Autodesk Inventor part; units mm, degrees
(part 2 of 2)
  spline S266 degree 2 poles (0.3678, -0.7093) (0.2402, -0.5675) (0.1065, -0.294) (0.1065, -0.14) knots 0 0 0 1 2 2 2
  spline S267 degree 2 poles (0.1065, -0.14) (0.1065, 0.1355) (0.4712, 0.4475) (0.8176, 0.4475) knots 0 0 0 1 2 2 2
  line L239 (0.8176, 0.4475) -> (2.0352, 0.4475)
  line L240 (2.831, -11.0699) -> (2.831, -12.2328)
  line L241 (2.831, -12.2328) -> (3.536, -12.2328)
  line L242 (3.536, -12.2328) -> (3.536, -11.1185)
  line L243 (3.536, -11.1185) -> (3.8318, -11.1185)
  line L244 (3.8318, -11.1185) -> (3.8318, -12.2328)
  line L245 (3.8318, -12.2328) -> (5.0352, -12.2328)
  line L246 (5.0352, -12.2328) -> (5.0352, -12.565)
  line L247 (5.0352, -12.565) -> (2.5352, -12.565)
  line L248 (2.5352, -12.565) -> (2.5352, -11.0699)
  line L249 (2.5352, -11.0699) -> (2.831, -11.0699)
  line L250 (5.0352, -10.4743) -> (5.0352, -10.7903)
  line L251 (5.0352, -10.7903) -> (3.1592, -10.7903)
  line L252 (3.1592, -10.7903) -> (3.1592, -10.4743)
  line L253 (3.1592, -10.4743) -> (5.0352, -10.4743)
  line L254 (2.8472, -10.452) -> (2.8472, -10.8106)
  line L255 (2.8472, -10.8106) -> (2.519, -10.8106)
  line L256 (2.519, -10.8106) -> (2.519, -10.452)
  line L257 (2.519, -10.452) -> (2.8472, -10.452)
  line L258 (5.0352, -9.6882) -> (5.0352, -10.0043)
  line L259 (5.0352, -10.0043) -> (2.4238, -10.0043)
  line L260 (2.4238, -10.0043) -> (2.4238, -9.6882)
  line L261 (2.4238, -9.6882) -> (5.0352, -9.6882)
  line L262 (5.0352, -8.9022) -> (5.0352, -9.2182)
  line L263 (5.0352, -9.2182) -> (3.1592, -9.2182)
  line L264 (3.1592, -9.2182) -> (3.1592, -8.9022)
  line L265 (3.1592, -8.9022) -> (5.0352, -8.9022)
  line L266 (2.8472, -8.8799) -> (2.8472, -9.2385)
  line L267 (2.8472, -9.2385) -> (2.519, -9.2385)
  line L268 (2.519, -9.2385) -> (2.519, -8.8799)
  line L269 (2.519, -8.8799) -> (2.8472, -8.8799)
  spline S268 degree 2 poles (4.0465, -6.8661) (4.5165, -6.8661) (5.0716, -7.3138) (5.0716, -7.6562) knots 0 0 0 1 2 2 2
  spline S269 degree 2 poles (5.0716, -7.6562) (5.0716, -7.796) (5.0068, -8.0108) (4.94, -8.1222) knots 0 0 0 1 2 2 2
  line L270 (4.94, -8.1222) -> (5.726, -8.1222)
  line L271 (5.726, -8.1222) -> (5.726, -8.4382)
  line L272 (5.726, -8.4382) -> (3.1592, -8.4382)
  line L273 (3.1592, -8.4382) -> (3.1592, -8.1222)
  line L274 (3.1592, -8.1222) -> (3.3557, -8.1222)
  spline S270 degree 2 poles (3.3557, -8.1222) (3.2483, -8.0047) (3.1065, -7.717) (3.1065, -7.5488) knots 0 0 0 1 2 2 2
  spline S271 degree 2 poles (3.1065, -7.5488) (3.1065, -7.2267) (3.617, -6.8661) (4.0465, -6.8661) knots 0 0 0 1 2 2 2
  spline S272 degree 2 poles (4.083, -7.1923) (3.7609, -7.1923) (3.4063, -7.3969) (3.4063, -7.6258) knots 0 0 0 1 2 2 2
  spline S273 degree 2 poles (3.4063, -7.6258) (3.4063, -7.7595) (3.5259, -8.0108) (3.6191, -8.1222) knots 0 0 0 1 2 2 2
  line L275 (3.6191, -8.1222) -> (4.6847, -8.1222)
  spline S274 degree 2 poles (4.6847, -8.1222) (4.7434, -7.9986) (4.788, -7.8223) (4.788, -7.7089) knots 0 0 0 1 2 2 2
  spline S275 degree 2 poles (4.788, -7.7089) (4.788, -7.4638) (4.4274, -7.1923) (4.083, -7.1923) knots 0 0 0 1 2 2 2
  line L276 (5.0352, -4.984) -> (5.0352, -5.3993)
  line L277 (5.0352, -5.3993) -> (4.1296, -6.0962)
  line L278 (4.1296, -6.0962) -> (4.2511, -6.2219)
  line L279 (4.2511, -6.2219) -> (5.0352, -6.2219)
  line L280 (5.0352, -6.2219) -> (5.0352, -6.5379)
  line L281 (5.0352, -6.5379) -> (2.4238, -6.5379)
  line L282 (2.4238, -6.5379) -> (2.4238, -6.2219)
  line L283 (2.4238, -6.2219) -> (3.9513, -6.2219)
  line L284 (3.9513, -6.2219) -> (3.1592, -5.4804)
  line L285 (3.1592, -5.4804) -> (3.1592, -5.0873)
  line L286 (3.1592, -5.0873) -> (3.9432, -5.8572)
  line L287 (3.9432, -5.8572) -> (5.0352, -4.984)
  spline S276 degree 2 poles (4.0972, -3.2843) (4.5712, -3.2843) (5.0879, -3.7401) (5.0879, -4.121) knots 0 0 0 1 2 2 2
  spline S277 degree 2 poles (5.0879, -4.121) (5.0879, -4.512) (4.555, -4.9597) (4.0972, -4.9597) knots 0 0 0 1 2 2 2
  spline S278 degree 2 poles (4.0972, -4.9597) (3.6272, -4.9597) (3.1065, -4.4978) (3.1065, -4.121) knots 0 0 0 1 2 2 2
  spline S279 degree 2 poles (3.1065, -4.121) (3.1065, -3.7401) (3.6251, -3.2843) (4.0972, -3.2843) knots 0 0 0 1 2 2 2
  spline S280 degree 2 poles (4.0972, -3.6104) (3.7325, -3.6104) (3.378, -3.8758) (3.378, -4.121) knots 0 0 0 1 2 2 2
  spline S281 degree 2 poles (3.378, -4.121) (3.378, -4.3661) (3.7325, -4.6335) (4.0972, -4.6335) knots 0 0 0 1 2 2 2
  spline S282 degree 2 poles (4.0972, -4.6335) (4.4517, -4.6335) (4.8164, -4.3661) (4.8164, -4.121) knots 0 0 0 1 2 2 2
  spline S283 degree 2 poles (4.8164, -4.121) (4.8164, -3.8779) (4.4578, -3.6104) (4.0972, -3.6104) knots 0 0 0 1 2 2 2
  line L288 (3.1592, -0.687) -> (5.0352, -1.1631)
  line L289 (5.0352, -1.1631) -> (5.0352, -1.4548)
  line L290 (5.0352, -1.4548) -> (3.5887, -1.9127)
  line L291 (3.5887, -1.9127) -> (5.0352, -2.3685)
  line L292 (5.0352, -2.3685) -> (5.0352, -2.6582)
  line L293 (5.0352, -2.6582) -> (3.1592, -3.1384)
  line L294 (3.1592, -3.1384) -> (3.1592, -2.8102)
  line L295 (3.1592, -2.8102) -> (4.6118, -2.4779)
  line L296 (4.6118, -2.4779) -> (3.1592, -2.0343)
  line L297 (3.1592, -2.0343) -> (3.1592, -1.7729)
  line L298 (3.1592, -1.7729) -> (4.6118, -1.3171)
  line L299 (4.6118, -1.3171) -> (3.1592, -1.0051)
  line L300 (3.1592, -1.0051) -> (3.1592, -0.687)
  spline S284 degree 2 poles (5.0797, 0.097) (5.0797, -0.0914) (4.9785, -0.4176) (4.9217, -0.5249) knots 0 0 0 1 2 2 2
  line L301 (4.9217, -0.5249) -> (4.5672, -0.5249)
  line L302 (4.5672, -0.5249) -> (4.5672, -0.5087)
  spline S285 degree 2 poles (4.5672, -0.5087) (4.5996, -0.4682) (4.6766, -0.3588) (4.7191, -0.2676) knots 0 0 0 1 2 2 2
  spline S286 degree 2 poles (4.7191, -0.2676) (4.7576, -0.1886) (4.8144, 0.0059) (4.8144, 0.1092) knots 0 0 0 1 2 2 2
  spline S287 degree 2 poles (4.8144, 0.1092) (4.8144, 0.1841) (4.7799, 0.3563) (4.7515, 0.3969) knots 0 0 0 1 2 2 2
  spline S288 degree 2 poles (4.7515, 0.3969) (4.7131, 0.4556) (4.6259, 0.5083) (4.5368, 0.5083) knots 0 0 0 1 2 2 2
  spline S289 degree 2 poles (4.5368, 0.5083) (4.4254, 0.5083) (4.3099, 0.3867) (4.2714, 0.2307) knots 0 0 0 1 2 2 2
  spline S290 degree 2 poles (4.2714, 0.2307) (4.2572, 0.17) (4.2167, -0.0245) (4.1944, -0.1076) knots 0 0 0 1 2 2 2
  spline S291 degree 2 poles (4.1944, -0.1076) (4.1316, -0.3223) (3.8723, -0.5168) (3.6879, -0.5168) knots 0 0 0 1 2 2 2
  spline S292 degree 2 poles (3.6879, -0.5168) (3.4327, -0.5168) (3.1146, -0.1339) (3.1146, 0.1821) knots 0 0 0 1 2 2 2
  spline S293 degree 2 poles (3.1146, 0.1821) (3.1146, 0.3381) (3.1916, 0.6542) (3.2503, 0.7615) knots 0 0 0 1 2 2 2
  line L303 (3.2503, 0.7615) -> (3.5887, 0.7615)
  line L304 (3.5887, 0.7615) -> (3.5887, 0.7453)
  spline S294 degree 2 poles (3.5887, 0.7453) (3.4914, 0.6238) (3.38, 0.328) (3.38, 0.176) knots 0 0 0 1 2 2 2
  spline S295 degree 2 poles (3.38, 0.176) (3.38, 0.02) (3.5117, -0.1947) (3.6434, -0.1947) knots 0 0 0 1 2 2 2
  spline S296 degree 2 poles (3.6434, -0.1947) (3.7629, -0.1947) (3.8784, -0.0671) (3.9148, 0.0747) knots 0 0 0 1 2 2 2
  spline S297 degree 2 poles (3.9148, 0.0747) (3.9331, 0.1436) (3.9695, 0.3179) (3.9918, 0.4131) knots 0 0 0 1 2 2 2
  spline S298 degree 2 poles (3.9918, 0.4131) (4.0445, 0.6197) (4.2856, 0.8304) (4.4943, 0.8304) knots 0 0 0 1 2 2 2
  spline S299 degree 2 poles (4.4943, 0.8304) (4.6158, 0.8304) (4.8306, 0.7352) (4.9096, 0.642) knots 0 0 0 1 2 2 2
  spline S300 degree 2 poles (4.9096, 0.642) (4.9926, 0.5427) (5.0797, 0.2895) (5.0797, 0.097) knots 0 0 0 1 2 2 2
  line L305 (5.0352, 2.6781) -> (5.0352, 2.2627)
  line L306 (5.0352, 2.2627) -> (4.1296, 1.5658)
  line L307 (4.1296, 1.5658) -> (4.2511, 1.4402)
  line L308 (4.2511, 1.4402) -> (5.0352, 1.4402)
  line L309 (5.0352, 1.4402) -> (5.0352, 1.1242)
  line L310 (5.0352, 1.1242) -> (2.4238, 1.1242)
  line L311 (2.4238, 1.1242) -> (2.4238, 1.4402)
  line L312 (2.4238, 1.4402) -> (3.9513, 1.4402)
  line L313 (3.9513, 1.4402) -> (3.1592, 2.1817)
  line L314 (3.1592, 2.1817) -> (3.1592, 2.5747)
  line L315 (3.1592, 2.5747) -> (3.9432, 1.8049)
  line L316 (3.9432, 1.8049) -> (5.0352, 2.6781)
  line L317 (5.0352, 3.1582) -> (5.0352, 2.8422)
  line L318 (5.0352, 2.8422) -> (3.1592, 2.8422)
  line L319 (3.1592, 2.8422) -> (3.1592, 3.1582)
  line L320 (3.1592, 3.1582) -> (5.0352, 3.1582)
  line L321 (2.8472, 3.1805) -> (2.8472, 2.8219)
  line L322 (2.8472, 2.8219) -> (2.519, 2.8219)
  line L323 (2.519, 2.8219) -> (2.519, 3.1805)
  line L324 (2.519, 3.1805) -> (2.8472, 3.1805)
  line L325 (10.2664, -10.4256) -> (10.2664, -10.8571)
  line L326 (10.2664, -10.8571) -> (9.2716, -11.6472)
  line L327 (9.2716, -11.6472) -> (9.2716, -12.0281)
  line L328 (9.2716, -12.0281) -> (10.2664, -12.0281)
  line L329 (10.2664, -12.0281) -> (10.2664, -12.3604)
  line L330 (10.2664, -12.3604) -> (7.7664, -12.3604)
  line L331 (7.7664, -12.3604) -> (7.7664, -11.7161)
  spline S301 degree 2 poles (7.7664, -11.7161) (7.7664, -11.5014) (7.8129, -11.2117) (7.898, -11.08) knots 0 0 0 1 2 2 2
  spline S302 degree 2 poles (7.898, -11.08) (7.9831, -10.9483) (8.2485, -10.7963) (8.445, -10.7963) knots 0 0 0 1 2 2 2
  spline S303 degree 2 poles (8.445, -10.7963) (8.7185, -10.7963) (9.0893, -11.0759) (9.1784, -11.315) knots 0 0 0 1 2 2 2
  line L332 (9.1784, -11.315) -> (10.2664, -10.4256)
  spline S304 degree 2 poles (8.4714, -11.1428) (8.362, -11.1428) (8.1938, -11.2198) (8.1391, -11.3008) knots 0 0 0 1 2 2 2
  spline S305 degree 2 poles (8.1391, -11.3008) (8.0925, -11.3717) (8.054, -11.5601) (8.054, -11.6979) knots 0 0 0 1 2 2 2
  line L333 (8.054, -11.6979) -> (8.054, -12.0281)
  line L334 (8.054, -12.0281) -> (8.9941, -12.0281)
  line L335 (8.9941, -12.0281) -> (8.9941, -11.7364)
  spline S306 degree 2 poles (8.9941, -11.7364) (8.9941, -11.5925) (8.9434, -11.3636) (8.8644, -11.2846) knots 0 0 0 1 2 2 2
  spline S307 degree 2 poles (8.8644, -11.2846) (8.7955, -11.2117) (8.601, -11.1428) (8.4714, -11.1428) knots 0 0 0 1 2 2 2
  spline S308 degree 2 poles (8.052, -8.4584) (8.2181, -8.3166) (8.7044, -8.1586) (9.0164, -8.1586) knots 0 0 0 1 2 2 2
  spline S309 degree 2 poles (9.0164, -8.1586) (9.3202, -8.1586) (9.8125, -8.3126) (9.9787, -8.4584) knots 0 0 0 1 2 2 2
  spline S310 degree 2 poles (9.9787, -8.4584) (10.1529, -8.6124) (10.319, -9.0196) (10.319, -9.2647) knots 0 0 0 1 2 2 2
  spline S311 degree 2 poles (10.319, -9.2647) (10.319, -9.518) (10.1468, -9.9232) (9.9787, -10.0711) knots 0 0 0 1 2 2 2
  spline S312 degree 2 poles (9.9787, -10.0711) (9.8125, -10.2149) (9.3243, -10.3689) (9.0164, -10.3689) knots 0 0 0 1 2 2 2
  spline S313 degree 2 poles (9.0164, -10.3689) (8.7023, -10.3689) (8.2242, -10.2129) (8.052, -10.069) knots 0 0 0 1 2 2 2
  spline S314 degree 2 poles (8.052, -10.069) (7.8859, -9.9232) (7.7137, -9.516) (7.7137, -9.2647) knots 0 0 0 1 2 2 2
  spline S315 degree 2 poles (7.7137, -9.2647) (7.7137, -9.0095) (7.892, -8.6002) (8.052, -8.4584) knots 0 0 0 1 2 2 2
  spline S316 degree 2 poles (9.0164, -8.505) (8.7692, -8.505) (8.3863, -8.6124) (8.2607, -8.7096) knots 0 0 0 1 2 2 2
  spline S317 degree 2 poles (8.2607, -8.7096) (8.131, -8.8089) (8.0014, -9.0885) (8.0014, -9.2627) knots 0 0 0 1 2 2 2
  spline S318 degree 2 poles (8.0014, -9.2627) (8.0014, -9.443) (8.127, -9.7145) (8.2607, -9.8178) knots 0 0 0 1 2 2 2
  spline S319 degree 2 poles (8.2607, -9.8178) (8.3883, -9.9171) (8.7732, -10.0224) (9.0164, -10.0224) knots 0 0 0 1 2 2 2
  spline S320 degree 2 poles (9.0164, -10.0224) (9.5087, -10.0224) (10.0313, -9.6092) (10.0313, -9.2627) knots 0 0 0 1 2 2 2
  spline S321 degree 2 poles (10.0313, -9.2627) (10.0313, -8.9163) (9.5087, -8.505) (9.0164, -8.505) knots 0 0 0 1 2 2 2
  spline S322 degree 2 poles (9.4985, -6.0982) (9.6849, -6.0982) (9.9706, -6.24) (10.0638, -6.3575) knots 0 0 0 1 2 2 2
  spline S323 degree 2 poles (10.0638, -6.3575) (10.1732, -6.4993) (10.2664, -6.8215) (10.2664, -7.0767) knots 0 0 0 1 2 2 2
  line L336 (10.2664, -7.0767) -> (10.2664, -7.7939)
  line L337 (10.2664, -7.7939) -> (7.7664, -7.7939)
  line L338 (7.7664, -7.7939) -> (7.7664, -7.1314)
  spline S324 degree 2 poles (7.7664, -7.1314) (7.7664, -6.864) (7.8008, -6.5966) (7.8676, -6.475) knots 0 0 0 1 2 2 2
  spline S325 degree 2 poles (7.8676, -6.475) (7.9386, -6.3393) (8.1715, -6.2157) (8.3296, -6.2157) knots 0 0 0 1 2 2 2
  spline S326 degree 2 poles (8.3296, -6.2157) (8.5058, -6.2157) (8.7854, -6.4021) (8.8644, -6.5662) knots 0 0 0 1 2 2 2
  line L339 (8.8644, -6.5662) -> (8.8766, -6.5662)
  spline S327 degree 2 poles (8.8766, -6.5662) (8.9373, -6.3433) (9.2595, -6.0982) (9.4985, -6.0982) knots 0 0 0 1 2 2 2
  spline S328 degree 2 poles (9.5127, -6.4446) (9.3709, -6.4446) (9.1886, -6.5257) (9.1237, -6.6472) knots 0 0 0 1 2 2 2
  spline S329 degree 2 poles (9.1237, -6.6472) (9.0832, -6.7263) (9.0589, -6.9126) (9.0589, -7.0848) knots 0 0 0 1 2 2 2
  line L340 (9.0589, -7.0848) -> (9.0589, -7.4617)
  line L341 (9.0589, -7.4617) -> (9.9827, -7.4617)
  line L342 (9.9827, -7.4617) -> (9.9827, -7.1922)
  spline S330 degree 2 poles (9.9827, -7.1922) (9.9827, -6.9734) (9.9422, -6.7222) (9.8774, -6.625) knots 0 0 0 1 2 2 2
  spline S331 degree 2 poles (9.8774, -6.625) (9.8105, -6.5318) (9.6444, -6.4446) (9.5127, -6.4446) knots 0 0 0 1 2 2 2
  spline S332 degree 2 poles (8.3762, -6.5622) (8.287, -6.5622) (8.1533, -6.6229) (8.1148, -6.6898) knots 0 0 0 1 2 2 2
  spline S333 degree 2 poles (8.1148, -6.6898) (8.0702, -6.7708) (8.05, -6.9673) (8.05, -7.1436) knots 0 0 0 1 2 2 2
  line L343 (8.05, -7.1436) -> (8.05, -7.4617)
  line L344 (8.05, -7.4617) -> (8.7813, -7.4617)
  line L345 (8.7813, -7.4617) -> (8.7813, -7.0848)
  spline S334 degree 2 poles (8.7813, -7.0848) (8.7813, -6.9288) (8.7489, -6.781) (8.6983, -6.7019) knots 0 0 0 1 2 2 2
  spline S335 degree 2 poles (8.6983, -6.7019) (8.6497, -6.625) (8.4937, -6.5622) (8.3762, -6.5622) knots 0 0 0 1 2 2 2
  spline S336 degree 2 poles (8.052, -3.9993) (8.2181, -3.8575) (8.7044, -3.6995) (9.0164, -3.6995) knots 0 0 0 1 2 2 2
  spline S337 degree 2 poles (9.0164, -3.6995) (9.3202, -3.6995) (9.8125, -3.8535) (9.9787, -3.9993) knots 0 0 0 1 2 2 2
  spline S338 degree 2 poles (9.9787, -3.9993) (10.1529, -4.1533) (10.319, -4.5605) (10.319, -4.8057) knots 0 0 0 1 2 2 2
  spline S339 degree 2 poles (10.319, -4.8057) (10.319, -5.0589) (10.1468, -5.4641) (9.9787, -5.612) knots 0 0 0 1 2 2 2
  spline S340 degree 2 poles (9.9787, -5.612) (9.8125, -5.7558) (9.3243, -5.9098) (9.0164, -5.9098) knots 0 0 0 1 2 2 2
  spline S341 degree 2 poles (9.0164, -5.9098) (8.7023, -5.9098) (8.2242, -5.7538) (8.052, -5.61) knots 0 0 0 1 2 2 2
  spline S342 degree 2 poles (8.052, -5.61) (7.8859, -5.4641) (7.7137, -5.0569) (7.7137, -4.8057) knots 0 0 0 1 2 2 2
  spline S343 degree 2 poles (7.7137, -4.8057) (7.7137, -4.5504) (7.892, -4.1412) (8.052, -3.9993) knots 0 0 0 1 2 2 2
  spline S344 degree 2 poles (9.0164, -4.0459) (8.7692, -4.0459) (8.3863, -4.1533) (8.2607, -4.2506) knots 0 0 0 1 2 2 2
  spline S345 degree 2 poles (8.2607, -4.2506) (8.131, -4.3498) (8.0014, -4.6294) (8.0014, -4.8036) knots 0 0 0 1 2 2 2
  spline S346 degree 2 poles (8.0014, -4.8036) (8.0014, -4.9839) (8.127, -5.2554) (8.2607, -5.3587) knots 0 0 0 1 2 2 2
  spline S347 degree 2 poles (8.2607, -5.3587) (8.3883, -5.458) (8.7732, -5.5634) (9.0164, -5.5634) knots 0 0 0 1 2 2 2
  spline S348 degree 2 poles (9.0164, -5.5634) (9.5087, -5.5634) (10.0313, -5.1501) (10.0313, -4.8036) knots 0 0 0 1 2 2 2
  spline S349 degree 2 poles (10.0313, -4.8036) (10.0313, -4.4572) (9.5087, -4.0459) (9.0164, -4.0459) knots 0 0 0 1 2 2 2
  line L346 (10.2664, -2.4637) -> (10.2664, -3.4321)
  line L347 (10.2664, -3.4321) -> (10.0111, -3.4321)
  line L348 (10.0111, -3.4321) -> (10.0111, -3.114)
  line L349 (10.0111, -3.114) -> (8.0216, -3.114)
  line L350 (8.0216, -3.114) -> (8.0216, -3.4321)
  line L351 (8.0216, -3.4321) -> (7.7664, -3.4321)
  line L352 (7.7664, -3.4321) -> (7.7664, -2.4637)
  line L353 (7.7664, -2.4637) -> (8.0216, -2.4637)
  line L354 (8.0216, -2.4637) -> (8.0216, -2.7818)
  line L355 (8.0216, -2.7818) -> (10.0111, -2.7818)
  line L356 (10.0111, -2.7818) -> (10.0111, -2.4637)
  line L357 (10.0111, -2.4637) -> (10.2664, -2.4637)
  line L358 (10.2664, -0.6039) -> (10.2664, -2.0524)
  line L359 (10.2664, -2.0524) -> (7.7664, -2.0524)
  line L360 (7.7664, -2.0524) -> (7.7664, -1.7202)
  line L361 (7.7664, -1.7202) -> (9.9706, -1.7202)
  line L362 (9.9706, -1.7202) -> (9.9706, -0.6039)
  line L363 (9.9706, -0.6039) -> (10.2664, -0.6039)
  spline S350 degree 2 poles (8.052, 1.4261) (8.2181, 1.5679) (8.7044, 1.7259) (9.0164, 1.7259) knots 0 0 0 1 2 2 2
  spline S351 degree 2 poles (9.0164, 1.7259) (9.3202, 1.7259) (9.8125, 1.572) (9.9787, 1.4261) knots 0 0 0 1 2 2 2
  spline S352 degree 2 poles (9.9787, 1.4261) (10.1529, 1.2721) (10.319, 0.8649) (10.319, 0.6198) knots 0 0 0 1 2 2 2
  spline S353 degree 2 poles (10.319, 0.6198) (10.319, 0.3665) (10.1468, -0.0386) (9.9787, -0.1865) knots 0 0 0 1 2 2 2
  spline S354 degree 2 poles (9.9787, -0.1865) (9.8125, -0.3304) (9.3243, -0.4844) (9.0164, -0.4844) knots 0 0 0 1 2 2 2
  spline S355 degree 2 poles (9.0164, -0.4844) (8.7023, -0.4844) (8.2242, -0.3284) (8.052, -0.1845) knots 0 0 0 1 2 2 2
  spline S356 degree 2 poles (8.052, -0.1845) (7.8859, -0.0386) (7.7137, 0.3686) (7.7137, 0.6198) knots 0 0 0 1 2 2 2
  spline S357 degree 2 poles (7.7137, 0.6198) (7.7137, 0.875) (7.892, 1.2843) (8.052, 1.4261) knots 0 0 0 1 2 2 2
  spline S358 degree 2 poles (9.0164, 1.3795) (8.7692, 1.3795) (8.3863, 1.2721) (8.2607, 1.1749) knots 0 0 0 1 2 2 2
  spline S359 degree 2 poles (8.2607, 1.1749) (8.131, 1.0756) (8.0014, 0.796) (8.0014, 0.6218) knots 0 0 0 1 2 2 2
  spline S360 degree 2 poles (8.0014, 0.6218) (8.0014, 0.4415) (8.127, 0.17) (8.2607, 0.0667) knots 0 0 0 1 2 2 2
  spline S361 degree 2 poles (8.2607, 0.0667) (8.3883, -0.0326) (8.7732, -0.1379) (9.0164, -0.1379) knots 0 0 0 1 2 2 2
  spline S362 degree 2 poles (9.0164, -0.1379) (9.5087, -0.1379) (10.0313, 0.2754) (10.0313, 0.6218) knots 0 0 0 1 2 2 2
  spline S363 degree 2 poles (10.0313, 0.6218) (10.0313, 0.9682) (9.5087, 1.3795) (9.0164, 1.3795) knots 0 0 0 1 2 2 2
  line L364 (6.5261, 13.9701) -> (6.5261, 13.5386)
  line L365 (6.5261, 13.5386) -> (5.5314, 12.7485)
  line L366 (5.5314, 12.7485) -> (5.5314, 12.3676)
  line L367 (5.5314, 12.3676) -> (6.5261, 12.3676)
  line L368 (6.5261, 12.3676) -> (6.5261, 12.0354)
  line L369 (6.5261, 12.0354) -> (4.0261, 12.0354)
  line L370 (4.0261, 12.0354) -> (4.0261, 12.6796)
  spline S364 degree 2 poles (4.0261, 12.6796) (4.0261, 12.8944) (4.0727, 13.1841) (4.1578, 13.3158) knots 0 0 0 1 2 2 2
  spline S365 degree 2 poles (4.1578, 13.3158) (4.2429, 13.4475) (4.5083, 13.5994) (4.7048, 13.5994) knots 0 0 0 1 2 2 2
  spline S366 degree 2 poles (4.7048, 13.5994) (4.9783, 13.5994) (5.349, 13.3198) (5.4382, 13.0808) knots 0 0 0 1 2 2 2
  line L371 (5.4382, 13.0808) -> (6.5261, 13.9701)
  spline S367 degree 2 poles (4.7311, 13.253) (4.6217, 13.253) (4.4536, 13.176) (4.3989, 13.0949) knots 0 0 0 1 2 2 2
  spline S368 degree 2 poles (4.3989, 13.0949) (4.3523, 13.024) (4.3138, 12.8356) (4.3138, 12.6979) knots 0 0 0 1 2 2 2
  line L372 (4.3138, 12.6979) -> (4.3138, 12.3676)
  line L373 (4.3138, 12.3676) -> (5.2538, 12.3676)
  line L374 (5.2538, 12.3676) -> (5.2538, 12.6594)
  spline S369 degree 2 poles (5.2538, 12.6594) (5.2538, 12.8032) (5.2032, 13.0321) (5.1242, 13.1111) knots 0 0 0 1 2 2 2
  spline S370 degree 2 poles (5.1242, 13.1111) (5.0553, 13.1841) (4.8608, 13.253) (4.7311, 13.253) knots 0 0 0 1 2 2 2
  line L375 (6.5261, 15.8968) -> (6.5261, 15.5159)
  line L376 (6.5261, 15.5159) -> (5.5294, 14.9082)
  line L377 (5.5294, 14.9082) -> (6.5261, 14.2882)
  line L378 (6.5261, 14.2882) -> (6.5261, 13.9296)
  line L379 (6.5261, 13.9296) -> (5.2741, 14.7258)
  line L380 (5.2741, 14.7258) -> (4.0261, 13.9539)
  line L381 (4.0261, 13.9539) -> (4.0261, 14.3348)
  line L382 (4.0261, 14.3348) -> (5.0046, 14.9304)
  line L383 (5.0046, 14.9304) -> (4.0261, 15.5382)
  line L384 (4.0261, 15.5382) -> (4.0261, 15.8968)
  line L385 (4.0261, 15.8968) -> (5.2579, 15.1148)
  line L386 (5.2579, 15.1148) -> (6.5261, 15.8968)
  line L387 (9.2261, 12.6817) -> (7.0219, 12.6817)
  line L388 (7.0219, 12.6817) -> (7.0219, 11.8429)
  line L389 (7.0219, 11.8429) -> (6.7261, 11.8429)
  line L390 (6.7261, 11.8429) -> (6.7261, 13.8526)
  line L391 (6.7261, 13.8526) -> (7.0219, 13.8526)
  line L392 (7.0219, 13.8526) -> (7.0219, 13.0139)
  line L393 (7.0219, 13.0139) -> (9.2261, 13.0139)
  line L394 (9.2261, 13.0139) -> (9.2261, 12.6817)
  line L395 (9.2261, 15.834) -> (9.2261, 15.4531)
  line L396 (9.2261, 15.4531) -> (8.2294, 14.8453)
  line L397 (8.2294, 14.8453) -> (9.2261, 14.2254)
  line L398 (9.2261, 14.2254) -> (9.2261, 13.8668)
  line L399 (9.2261, 13.8668) -> (7.9741, 14.663)
  line L400 (7.9741, 14.663) -> (6.7261, 13.8911)
  line L401 (6.7261, 13.8911) -> (6.7261, 14.272)
  line L402 (6.7261, 14.272) -> (7.7046, 14.8676)
  line L403 (7.7046, 14.8676) -> (6.7261, 15.4754)
  line L404 (6.7261, 15.4754) -> (6.7261, 15.834)
  line L405 (6.7261, 15.834) -> (7.9579, 15.052)
  line L406 (7.9579, 15.052) -> (9.2261, 15.834)
  spline S371 degree 2 poles (11.9747, 11.6859) (11.9747, 11.4205) (11.8127, 10.9809) (11.6486, 10.8229) knots 0 0 0 1 2 2 2
  spline S372 degree 2 poles (11.6486, 10.8229) (11.4824, 10.6648) (10.9922, 10.4967) (10.6741, 10.4967) knots 0 0 0 1 2 2 2
  spline S373 degree 2 poles (10.6741, 10.4967) (10.3722, 10.4967) (9.8941, 10.6669) (9.7239, 10.8249) knots 0 0 0 1 2 2 2
  spline S374 degree 2 poles (9.7239, 10.8249) (9.5598, 10.9768) (9.3815, 11.4225) (9.3815, 11.6879) knots 0 0 0 1 2 2 2
  spline S375 degree 2 poles (9.3815, 11.6879) (9.3815, 11.8156) (9.418, 12.0465) (9.4504, 12.1519) knots 0 0 0 1 2 2 2
  spline S376 degree 2 poles (9.4504, 12.1519) (9.4747, 12.237) (9.5639, 12.4436) (9.5963, 12.5064) knots 0 0 0 1 2 2 2
  line L407 (9.5963, 12.5064) -> (9.9974, 12.5064)
  line L408 (9.9974, 12.5064) -> (9.9974, 12.478)
  spline S377 degree 2 poles (9.9974, 12.478) (9.9427, 12.4152) (9.8435, 12.2836) (9.7867, 12.162) knots 0 0 0 1 2 2 2
  spline S378 degree 2 poles (9.7867, 12.162) (9.7361, 12.0607) (9.6692, 11.7994) (9.6692, 11.6494) knots 0 0 0 1 2 2 2
  spline S379 degree 2 poles (9.6692, 11.6494) (9.6692, 11.2888) (10.2122, 10.8431) (10.664, 10.8431) knots 0 0 0 1 2 2 2
  spline S380 degree 2 poles (10.664, 10.8431) (10.9152, 10.8431) (11.292, 10.9606) (11.4217, 11.072) knots 0 0 0 1 2 2 2
  spline S381 degree 2 poles (11.4217, 11.072) (11.5513, 11.1794) (11.687, 11.4833) (11.687, 11.6738) knots 0 0 0 1 2 2 2
  spline S382 degree 2 poles (11.687, 11.6738) (11.687, 11.8135) (11.6465, 12.0931) (11.606, 12.1883) knots 0 0 0 1 2 2 2
  line L409 (11.606, 12.1883) -> (10.9597, 12.1883)
  line L410 (10.9597, 12.1883) -> (10.9597, 11.6089)
  line L411 (10.9597, 11.6089) -> (10.668, 11.6089)
  line L412 (10.668, 11.6089) -> (10.668, 12.5165)
  line L413 (10.668, 12.5165) -> (11.76, 12.5165)
  spline S383 degree 2 poles (11.76, 12.5165) (11.7883, 12.4537) (11.8755, 12.239) (11.9018, 12.1478) knots 0 0 0 1 2 2 2
  spline S384 degree 2 poles (11.9018, 12.1478) (11.9383, 12.0242) (11.9747, 11.8257) (11.9747, 11.6859) knots 0 0 0 1 2 2 2
  line L414 (11.9261, 14.7228) -> (11.9261, 14.35)
  line L415 (11.9261, 14.35) -> (9.7705, 13.2438)
  line L416 (9.7705, 13.2438) -> (11.9261, 13.2438)
  line L417 (11.9261, 13.2438) -> (11.9261, 12.9339)
  line L418 (11.9261, 12.9339) -> (9.4261, 12.9339)
  line L419 (9.4261, 12.9339) -> (9.4261, 13.4059)
  line L420 (9.4261, 13.4059) -> (11.4054, 14.4128)
  line L421 (11.4054, 14.4128) -> (9.4261, 14.4128)
  line L422 (9.4261, 14.4128) -> (9.4261, 14.7228)
  line L423 (9.4261, 14.7228) -> (11.9261, 14.7228)
  spline S385 degree 2 poles (10.6781, 17.2005) (11.0205, 17.2005) (11.5716, 16.9229) (11.7255, 16.69) knots 0 0 0 1 2 2 2
  spline S386 degree 2 poles (11.7255, 16.69) (11.8451, 16.4995) (11.9261, 16.1085) (11.9261, 15.8046) knots 0 0 0 1 2 2 2
  line L424 (11.9261, 15.8046) -> (11.9261, 15.2293)
  line L425 (11.9261, 15.2293) -> (9.4261, 15.2293)
  line L426 (9.4261, 15.2293) -> (9.4261, 15.7985)
  spline S387 degree 2 poles (9.4261, 15.7985) (9.4261, 16.1511) (9.5315, 16.5522) (9.6247, 16.694) knots 0 0 0 1 2 2 2
  spline S388 degree 2 poles (9.6247, 16.694) (9.7847, 16.9351) (10.3135, 17.2005) (10.6781, 17.2005) knots 0 0 0 1 2 2 2
  spline S389 degree 2 poles (10.6741, 16.8541) (10.3864, 16.8541) (9.9792, 16.6636) (9.8637, 16.4752) knots 0 0 0 1 2 2 2
  spline S390 degree 2 poles (9.8637, 16.4752) (9.7847, 16.3415) (9.7138, 16.0396) (9.7138, 15.8148) knots 0 0 0 1 2 2 2
  line L427 (9.7138, 15.8148) -> (9.7138, 15.5615)
  line L428 (9.7138, 15.5615) -> (11.6384, 15.5615)
  line L429 (11.6384, 15.5615) -> (11.6384, 15.8148)
  spline S391 degree 2 poles (11.6384, 15.8148) (11.6384, 16.0356) (11.5675, 16.3699) (11.4723, 16.5056) knots 0 0 0 1 2 2 2
  spline S392 degree 2 poles (11.4723, 16.5056) (11.3548, 16.6798) (10.9658, 16.8541) (10.6741, 16.8541) knots 0 0 0 1 2 2 2
  line L430 (-4.6376, 12.4989) -> (-4.6376, 12.1667)
  line L431 (-4.6376, 12.1667) -> (-6.7912, 12.1667)
  line L432 (-6.7912, 12.1667) -> (-5.3264, 11.5143)
  line L433 (-5.3264, 11.5143) -> (-5.3264, 11.3117)
  line L434 (-5.3264, 11.3117) -> (-6.7912, 10.6655)
  line L435 (-6.7912, 10.6655) -> (-4.6376, 10.6655)
  line L436 (-4.6376, 10.6655) -> (-4.6376, 10.3555)
  line L437 (-4.6376, 10.3555) -> (-7.1376, 10.3555)
  line L438 (-7.1376, 10.3555) -> (-7.1376, 10.8093)
  line L439 (-7.1376, 10.8093) -> (-5.7458, 11.4333)
  line L440 (-5.7458, 11.4333) -> (-7.1376, 12.037)
  line L441 (-7.1376, 12.037) -> (-7.1376, 12.4989)
  line L442 (-7.1376, 12.4989) -> (-4.6376, 12.4989)
  spline S393 degree 2 poles (-6.8519, 14.774) (-6.6858, 14.9159) (-6.1996, 15.0739) (-5.8876, 15.0739) knots 0 0 0 1 2 2 2
  spline S394 degree 2 poles (-5.8876, 15.0739) (-5.5837, 15.0739) (-5.0914, 14.9199) (-4.9253, 14.774) knots 0 0 0 1 2 2 2
  spline S395 degree 2 poles (-4.9253, 14.774) (-4.751, 14.6201) (-4.5849, 14.2129) (-4.5849, 13.9677) knots 0 0 0 1 2 2 2
  spline S396 degree 2 poles (-4.5849, 13.9677) (-4.5849, 13.7145) (-4.7571, 13.3093) (-4.9253, 13.1614) knots 0 0 0 1 2 2 2
  spline S397 degree 2 poles (-4.9253, 13.1614) (-5.0914, 13.0176) (-5.5796, 12.8636) (-5.8876, 12.8636) knots 0 0 0 1 2 2 2
  spline S398 degree 2 poles (-5.8876, 12.8636) (-6.2016, 12.8636) (-6.6797, 13.0196) (-6.8519, 13.1634) knots 0 0 0 1 2 2 2
  spline S399 degree 2 poles (-6.8519, 13.1634) (-7.0181, 13.3093) (-7.1903, 13.7165) (-7.1903, 13.9677) knots 0 0 0 1 2 2 2
  spline S400 degree 2 poles (-7.1903, 13.9677) (-7.1903, 14.223) (-7.012, 14.6322) (-6.8519, 14.774) knots 0 0 0 1 2 2 2
  spline S401 degree 2 poles (-5.8876, 14.7274) (-6.1348, 14.7274) (-6.5177, 14.6201) (-6.6433, 14.5228) knots 0 0 0 1 2 2 2
  spline S402 degree 2 poles (-6.6433, 14.5228) (-6.7729, 14.4236) (-6.9026, 14.144) (-6.9026, 13.9698) knots 0 0 0 1 2 2 2
  spline S403 degree 2 poles (-6.9026, 13.9698) (-6.9026, 13.7894) (-6.777, 13.518) (-6.6433, 13.4146) knots 0 0 0 1 2 2 2
  spline S404 degree 2 poles (-6.6433, 13.4146) (-6.5156, 13.3154) (-6.1307, 13.21) (-5.8876, 13.21) knots 0 0 0 1 2 2 2
  spline S405 degree 2 poles (-5.8876, 13.21) (-5.3953, 13.21) (-4.8726, 13.6233) (-4.8726, 13.9698) knots 0 0 0 1 2 2 2
  spline S406 degree 2 poles (-4.8726, 13.9698) (-4.8726, 14.3162) (-5.3953, 14.7274) (-5.8876, 14.7274) knots 0 0 0 1 2 2 2
  spline S407 degree 2 poles (-5.8856, 17.4098) (-5.5432, 17.4098) (-4.9921, 17.1322) (-4.8382, 16.8992) knots 0 0 0 1 2 2 2
  spline S408 degree 2 poles (-4.8382, 16.8992) (-4.7186, 16.7088) (-4.6376, 16.3178) (-4.6376, 16.0139) knots 0 0 0 1 2 2 2
  line L443 (-4.6376, 16.0139) -> (-4.6376, 15.4386)
  line L444 (-4.6376, 15.4386) -> (-7.1376, 15.4386)
  line L445 (-7.1376, 15.4386) -> (-7.1376, 16.0078)
  spline S409 degree 2 poles (-7.1376, 16.0078) (-7.1376, 16.3604) (-7.0322, 16.7615) (-6.939, 16.9033) knots 0 0 0 1 2 2 2
  spline S410 degree 2 poles (-6.939, 16.9033) (-6.779, 17.1444) (-6.2502, 17.4098) (-5.8856, 17.4098) knots 0 0 0 1 2 2 2
  spline S411 degree 2 poles (-5.8896, 17.0633) (-6.1773, 17.0633) (-6.5845, 16.8729) (-6.7, 16.6845) knots 0 0 0 1 2 2 2
  spline S412 degree 2 poles (-6.7, 16.6845) (-6.779, 16.5508) (-6.8499, 16.2489) (-6.8499, 16.024) knots 0 0 0 1 2 2 2
  line L446 (-6.8499, 16.024) -> (-6.8499, 15.7708)
  line L447 (-6.8499, 15.7708) -> (-4.9253, 15.7708)
  line L448 (-4.9253, 15.7708) -> (-4.9253, 16.024)
  spline S413 degree 2 poles (-4.9253, 16.024) (-4.9253, 16.2449) (-4.9962, 16.5792) (-5.0914, 16.7149) knots 0 0 0 1 2 2 2
  spline S414 degree 2 poles (-5.0914, 16.7149) (-5.2089, 16.8891) (-5.5979, 17.0633) (-5.8896, 17.0633) knots 0 0 0 1 2 2 2
  line L449 (-1.9376, 13.1452) -> (-1.9376, 12.1768)
  line L450 (-1.9376, 12.1768) -> (-2.1929, 12.1768)
  line L451 (-2.1929, 12.1768) -> (-2.1929, 12.4949)
  line L452 (-2.1929, 12.4949) -> (-4.1823, 12.4949)
  line L453 (-4.1823, 12.4949) -> (-4.1823, 12.1768)
  line L454 (-4.1823, 12.1768) -> (-4.4376, 12.1768)
  line L455 (-4.4376, 12.1768) -> (-4.4376, 13.1452)
  line L456 (-4.4376, 13.1452) -> (-4.1823, 13.1452)
  line L457 (-4.1823, 13.1452) -> (-4.1823, 12.8271)
  line L458 (-4.1823, 12.8271) -> (-2.1929, 12.8271)
  line L459 (-2.1929, 12.8271) -> (-2.1929, 13.1452)
  line L460 (-2.1929, 13.1452) -> (-1.9376, 13.1452)
  line L461 (-1.9376, 15.3454) -> (-1.9376, 14.9726)
  line L462 (-1.9376, 14.9726) -> (-4.0932, 13.8664)
  line L463 (-4.0932, 13.8664) -> (-1.9376, 13.8664)
  line L464 (-1.9376, 13.8664) -> (-1.9376, 13.5565)
  line L465 (-1.9376, 13.5565) -> (-4.4376, 13.5565)
  line L466 (-4.4376, 13.5565) -> (-4.4376, 14.0285)
  line L467 (-4.4376, 14.0285) -> (-2.4583, 15.0354)
  line L468 (-2.4583, 15.0354) -> (-4.4376, 15.0354)
  line L469 (-4.4376, 15.0354) -> (-4.4376, 15.3454)
  line L470 (-4.4376, 15.3454) -> (-1.9376, 15.3454)
  spline S415 degree 2 poles (0.811, 11.649) (0.811, 11.3836) (0.649, 10.944) (0.4849, 10.786) knots 0 0 0 1 2 2 2
  spline S416 degree 2 poles (0.4849, 10.786) (0.3187, 10.628) (-0.1715, 10.4598) (-0.4896, 10.4598) knots 0 0 0 1 2 2 2
  spline S417 degree 2 poles (-0.4896, 10.4598) (-0.7915, 10.4598) (-1.2696, 10.63) (-1.4398, 10.788) knots 0 0 0 1 2 2 2
  spline S418 degree 2 poles (-1.4398, 10.788) (-1.6039, 10.94) (-1.7822, 11.3857) (-1.7822, 11.6511) knots 0 0 0 1 2 2 2
  spline S419 degree 2 poles (-1.7822, 11.6511) (-1.7822, 11.7787) (-1.7457, 12.0097) (-1.7133, 12.115) knots 0 0 0 1 2 2 2
  spline S420 degree 2 poles (-1.7133, 12.115) (-1.689, 12.2001) (-1.5998, 12.4067) (-1.5674, 12.4695) knots 0 0 0 1 2 2 2
  line L471 (-1.5674, 12.4695) -> (-1.1663, 12.4695)
  line L472 (-1.1663, 12.4695) -> (-1.1663, 12.4412)
  spline S421 degree 2 poles (-1.1663, 12.4412) (-1.221, 12.3784) (-1.3202, 12.2467) (-1.377, 12.1251) knots 0 0 0 1 2 2 2
  spline S422 degree 2 poles (-1.377, 12.1251) (-1.4276, 12.0238) (-1.4945, 11.7625) (-1.4945, 11.6126) knots 0 0 0 1 2 2 2
  spline S423 degree 2 poles (-1.4945, 11.6126) (-1.4945, 11.252) (-0.9515, 10.8063) (-0.4997, 10.8063) knots 0 0 0 1 2 2 2
  spline S424 degree 2 poles (-0.4997, 10.8063) (-0.2485, 10.8063) (0.1283, 10.9238) (0.258, 11.0352) knots 0 0 0 1 2 2 2
  spline S425 degree 2 poles (0.258, 11.0352) (0.3876, 11.1426) (0.5234, 11.4465) (0.5234, 11.6369) knots 0 0 0 1 2 2 2
  spline S426 degree 2 poles (0.5234, 11.6369) (0.5234, 11.7767) (0.4828, 12.0563) (0.4423, 12.1515) knots 0 0 0 1 2 2 2
  line L473 (0.4423, 12.1515) -> (-0.204, 12.1515)
  line L474 (-0.204, 12.1515) -> (-0.204, 11.5721)
  line L475 (-0.204, 11.5721) -> (-0.4957, 11.5721)
  line L476 (-0.4957, 11.5721) -> (-0.4957, 12.4797)
  line L477 (-0.4957, 12.4797) -> (0.5963, 12.4797)
  spline S427 degree 2 poles (0.5963, 12.4797) (0.6246, 12.4169) (0.7118, 12.2021) (0.7381, 12.111) knots 0 0 0 1 2 2 2
  spline S428 degree 2 poles (0.7381, 12.111) (0.7746, 11.9874) (0.811, 11.7888) (0.811, 11.649) knots 0 0 0 1 2 2 2
  line L478 (0.7624, 14.6859) -> (0.7624, 14.3131)
  line L479 (0.7624, 14.3131) -> (-1.3932, 13.207)
  line L480 (-1.3932, 13.207) -> (0.7624, 13.207)
  line L481 (0.7624, 13.207) -> (0.7624, 12.897)
  line L482 (0.7624, 12.897) -> (-1.7376, 12.897)
  line L483 (-1.7376, 12.897) -> (-1.7376, 13.3691)
  line L484 (-1.7376, 13.3691) -> (0.2417, 14.376)
  line L485 (0.2417, 14.376) -> (-1.7376, 14.376)
  line L486 (-1.7376, 14.376) -> (-1.7376, 14.6859)
  line L487 (-1.7376, 14.6859) -> (0.7624, 14.6859)
  spline S429 degree 2 poles (-0.4856, 17.1636) (-0.1432, 17.1636) (0.4079, 16.8861) (0.5618, 16.6531) knots 0 0 0 1 2 2 2
  spline S430 degree 2 poles (0.5618, 16.6531) (0.6814, 16.4627) (0.7624, 16.0717) (0.7624, 15.7678) knots 0 0 0 1 2 2 2
  line L488 (0.7624, 15.7678) -> (0.7624, 15.1924)
  line L489 (0.7624, 15.1924) -> (-1.7376, 15.1924)
  line L490 (-1.7376, 15.1924) -> (-1.7376, 15.7617)
  spline S431 degree 2 poles (-1.7376, 15.7617) (-1.7376, 16.1142) (-1.6322, 16.5153) (-1.539, 16.6571) knots 0 0 0 1 2 2 2
  spline S432 degree 2 poles (-1.539, 16.6571) (-1.379, 16.8982) (-0.8502, 17.1636) (-0.4856, 17.1636) knots 0 0 0 1 2 2 2
  spline S433 degree 2 poles (-0.4896, 16.8172) (-0.7773, 16.8172) (-1.1845, 16.6268) (-1.3, 16.4383) knots 0 0 0 1 2 2 2
  spline S434 degree 2 poles (-1.3, 16.4383) (-1.379, 16.3046) (-1.4499, 16.0028) (-1.4499, 15.7779) knots 0 0 0 1 2 2 2
  line L491 (-1.4499, 15.7779) -> (-1.4499, 15.5247)
  line L492 (-1.4499, 15.5247) -> (0.4747, 15.5247)
  line L493 (0.4747, 15.5247) -> (0.4747, 15.7779)
  spline S435 degree 2 poles (0.4747, 15.7779) (0.4747, 15.9987) (0.4038, 16.333) (0.3086, 16.4687) knots 0 0 0 1 2 2 2
  spline S436 degree 2 poles (0.3086, 16.4687) (0.1911, 16.643) (-0.1979, 16.8172) (-0.4896, 16.8172) knots 0 0 0 1 2 2 2
  spline S437 degree 2 poles (1.1994, 11.414) (1.1994, 11.3229) (1.244, 11.1426) (1.2785, 11.0554) knots 0 0 0 1 2 2 2
  spline S438 degree 2 poles (1.2785, 11.0554) (1.3129, 10.9744) (1.3858, 10.8549) (1.4182, 10.8083) knots 0 0 0 1 2 2 2
  line L494 (1.4182, 10.8083) -> (1.4182, 10.788)
  line L495 (1.4182, 10.788) -> (1.0637, 10.788)
  spline S439 degree 2 poles (1.0637, 10.788) (1.005, 10.8974) (0.9097, 11.2722) (0.9097, 11.4404) knots 0 0 0 1 2 2 2
  spline S440 degree 2 poles (0.9097, 11.4404) (0.9097, 11.6106) (0.9786, 11.8638) (1.0516, 11.9671) knots 0 0 0 1 2 2 2
  spline S441 degree 2 poles (1.0516, 11.9671) (1.1306, 12.0765) (1.3595, 12.19) (1.5135, 12.19) knots 0 0 0 1 2 2 2
  spline S442 degree 2 poles (1.5135, 12.19) (1.7201, 12.19) (2.0321, 11.9185) (2.0726, 11.7281) knots 0 0 0 1 2 2 2
  line L496 (2.0726, 11.7281) -> (2.0969, 11.7281)
  spline S443 degree 2 poles (2.0969, 11.7281) (2.1131, 11.8071) (2.1861, 11.9874) (2.259, 12.0644) knots 0 0 0 1 2 2 2
  spline S444 degree 2 poles (2.259, 12.0644) (2.3299, 12.1413) (2.5568, 12.2386) (2.7209, 12.2386) knots 0 0 0 1 2 2 2
  spline S445 degree 2 poles (2.7209, 12.2386) (2.8891, 12.2386) (3.1747, 12.1231) (3.2841, 12.0178) knots 0 0 0 1 2 2 2
  spline S446 degree 2 poles (3.2841, 12.0178) (3.3976, 11.9084) (3.5151, 11.5984) (3.5151, 11.4019) knots 0 0 0 1 2 2 2
  spline S447 degree 2 poles (3.5151, 11.4019) (3.5151, 11.2135) (3.4239, 10.8448) (3.3611, 10.7191) knots 0 0 0 1 2 2 2
  line L497 (3.3611, 10.7191) -> (3.0066, 10.7191)
  line L498 (3.0066, 10.7191) -> (3.0066, 10.7435)
  spline S448 degree 2 poles (3.0066, 10.7435) (3.0836, 10.8488) (3.2254, 11.2054) (3.2254, 11.3816) knots 0 0 0 1 2 2 2
  spline S449 degree 2 poles (3.2254, 11.3816) (3.2254, 11.4849) (3.1605, 11.6916) (3.0856, 11.7605) knots 0 0 0 1 2 2 2
  spline S450 degree 2 poles (3.0856, 11.7605) (3.0106, 11.8273) (2.8323, 11.8982) (2.6966, 11.8982) knots 0 0 0 1 2 2 2
  spline S451 degree 2 poles (2.6966, 11.8982) (2.5609, 11.8982) (2.3846, 11.8192) (2.334, 11.7483) knots 0 0 0 1 2 2 2
  spline S452 degree 2 poles (2.334, 11.7483) (2.2833, 11.6774) (2.2448, 11.4849) (2.2448, 11.3715) knots 0 0 0 1 2 2 2
  line L499 (2.2448, 11.3715) -> (2.2448, 11.2297)
  line L500 (2.2448, 11.2297) -> (1.9673, 11.2297)
  line L501 (1.9673, 11.2297) -> (1.9673, 11.3411)
  spline S453 degree 2 poles (1.9673, 11.3411) (1.9673, 11.566) (1.7525, 11.8496) (1.5479, 11.8496) knots 0 0 0 1 2 2 2
  spline S454 degree 2 poles (1.5479, 11.8496) (1.4527, 11.8496) (1.3169, 11.7767) (1.2764, 11.7179) knots 0 0 0 1 2 2 2
  spline S455 degree 2 poles (1.2764, 11.7179) (1.2339, 11.6551) (1.1994, 11.5012) (1.1994, 11.414) knots 0 0 0 1 2 2 2
  line L502 (3.4624, 13.1523) -> (3.4624, 12.7512)
  line L503 (3.4624, 12.7512) -> (2.9843, 12.7512)
  line L504 (2.9843, 12.7512) -> (2.9843, 13.1523)
  line L505 (2.9843, 13.1523) -> (3.4624, 13.1523)
  spline S456 degree 2 poles (1.1994, 14.3314) (1.1994, 14.2402) (1.244, 14.0599) (1.2785, 13.9728) knots 0 0 0 1 2 2 2
  spline S457 degree 2 poles (1.2785, 13.9728) (1.3129, 13.8918) (1.3858, 13.7722) (1.4182, 13.7256) knots 0 0 0 1 2 2 2
  line L506 (1.4182, 13.7256) -> (1.4182, 13.7054)
  line L507 (1.4182, 13.7054) -> (1.0637, 13.7054)
  spline S458 degree 2 poles (1.0637, 13.7054) (1.005, 13.8148) (0.9097, 14.1896) (0.9097, 14.3577) knots 0 0 0 1 2 2 2
  spline S459 degree 2 poles (0.9097, 14.3577) (0.9097, 14.5279) (0.9786, 14.7811) (1.0516, 14.8845) knots 0 0 0 1 2 2 2
  spline S460 degree 2 poles (1.0516, 14.8845) (1.1306, 14.9939) (1.3595, 15.1073) (1.5135, 15.1073) knots 0 0 0 1 2 2 2
  spline S461 degree 2 poles (1.5135, 15.1073) (1.7201, 15.1073) (2.0321, 14.8358) (2.0726, 14.6454) knots 0 0 0 1 2 2 2
  line L508 (2.0726, 14.6454) -> (2.0969, 14.6454)
  spline S462 degree 2 poles (2.0969, 14.6454) (2.1131, 14.7244) (2.1861, 14.9047) (2.259, 14.9817) knots 0 0 0 1 2 2 2
  spline S463 degree 2 poles (2.259, 14.9817) (2.3299, 15.0587) (2.5568, 15.1559) (2.7209, 15.1559) knots 0 0 0 1 2 2 2
  spline S464 degree 2 poles (2.7209, 15.1559) (2.8891, 15.1559) (3.1747, 15.0405) (3.2841, 14.9351) knots 0 0 0 1 2 2 2
  spline S465 degree 2 poles (3.2841, 14.9351) (3.3976, 14.8257) (3.5151, 14.5157) (3.5151, 14.3192) knots 0 0 0 1 2 2 2
  spline S466 degree 2 poles (3.5151, 14.3192) (3.5151, 14.1308) (3.4239, 13.7621) (3.3611, 13.6365) knots 0 0 0 1 2 2 2
  line L509 (3.3611, 13.6365) -> (3.0066, 13.6365)
  line L510 (3.0066, 13.6365) -> (3.0066, 13.6608)
  spline S467 degree 2 poles (3.0066, 13.6608) (3.0836, 13.7661) (3.2254, 14.1227) (3.2254, 14.299) knots 0 0 0 1 2 2 2
  spline S468 degree 2 poles (3.2254, 14.299) (3.2254, 14.4023) (3.1605, 14.6089) (3.0856, 14.6778) knots 0 0 0 1 2 2 2
  spline S469 degree 2 poles (3.0856, 14.6778) (3.0106, 14.7447) (2.8323, 14.8156) (2.6966, 14.8156) knots 0 0 0 1 2 2 2
  spline S470 degree 2 poles (2.6966, 14.8156) (2.5609, 14.8156) (2.3846, 14.7366) (2.334, 14.6657) knots 0 0 0 1 2 2 2
  spline S471 degree 2 poles (2.334, 14.6657) (2.2833, 14.5948) (2.2448, 14.4023) (2.2448, 14.2888) knots 0 0 0 1 2 2 2
  line L511 (2.2448, 14.2888) -> (2.2448, 14.147)
  line L512 (2.2448, 14.147) -> (1.9673, 14.147)
  line L513 (1.9673, 14.147) -> (1.9673, 14.2584)
  spline S472 degree 2 poles (1.9673, 14.2584) (1.9673, 14.4833) (1.7525, 14.767) (1.5479, 14.767) knots 0 0 0 1 2 2 2
  spline S473 degree 2 poles (1.5479, 14.767) (1.4527, 14.767) (1.3169, 14.694) (1.2764, 14.6353) knots 0 0 0 1 2 2 2
  spline S474 degree 2 poles (1.2764, 14.6353) (1.2339, 14.5725) (1.1994, 14.4185) (1.1994, 14.3314) knots 0 0 0 1 2 2 2
  line L514 (1.5864, 17.0522) -> (3.4624, 16.3452)
  line L515 (3.4624, 16.3452) -> (3.4624, 16.0615)
  line L516 (3.4624, 16.0615) -> (1.5864, 15.3606)
  line L517 (1.5864, 15.3606) -> (1.5864, 15.7029)
  line L518 (1.5864, 15.7029) -> (3.0309, 16.2155)
  line L519 (3.0309, 16.2155) -> (1.5864, 16.724)
  line L520 (1.5864, 16.724) -> (1.5864, 17.0522)
  point P0 (0, 0)
  constraints: 12 other
extrude "Extrusion2" add sketch "Sketch2" along normal blind 0.5
fillet "Fillet2" radius 1 4 edges at (-13.0046, 19.6218, 0.4) (-13.0046, -19.6218, 0.4) (13.0139, -19.6218, 0.4) (13.0139, 19.6218, 0.4)
body "Solid1"
